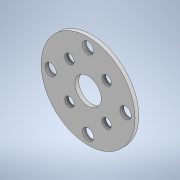
# Autodesk Inventor part: holes
Saved by Autodesk Inventor 2021.5 (Build 255421000, 421)
## iProperties
Created: 2024-11-26
Part Number: holes
Material: Genérico
Document SubType Name: Modeling
Designer: Joho_
Density: 1 g/cm^3
Appearance: Valor por defecto
Author: Joho_
## iProperties of the stored document _3DPrint.ipt
Created: 2024-11-26
Part Number: _3DPrint
Material: Genérico
Document SubType Name: Modeling
Designer: Joho_
Density: 1 g/cm^3
Appearance: Valor por defecto
Author: Joho_
Autodesk Inventor part; units mm, degrees
ref_plane "YZ Plane" through (0, 0, 0) normal (1, 0, 0) x (0, 1, 0)
ref_plane "XZ Plane" through (0, 0, 0) normal (0, 1, 0) x (-1, 0, 0)
ref_plane "XY Plane" through (0, 0, 0) normal (0, 0, 1) x (1, 0, 0)
sketch "Boceto1" plane through (0, 0, 0) normal (0, 0, 1) x (1, 0, 0)
  circle A0 centre (-9.9038, -9.9038) radius 2.5
  circle A1 centre (-9.9038, 9.9038) radius 2.5
  circle A2 centre (-20, 0) radius 3
  circle A3 centre (0, 20) radius 3
  circle A4 centre (20, 0) radius 3
  circle A5 centre (0, -20) radius 3
  circle A6 centre (0, 0) radius 25
  circle A7 centre (0, 0) radius 7
  circle A8 centre (9.9038, 9.9038) radius 2.5
  circle A9 centre (9.9038, -9.9038) radius 2.5
  constraints: 19 centre point
extrude "Extrusión1" add sketch "Boceto1" along normal blind 2
